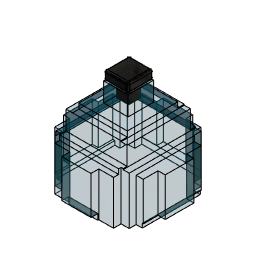
Sans nom v2 (Autodesk Fusion 360 design; units mm, degrees)
Autodesk Fusion 360 part; units mm, degrees
sketch "Esquisse1" plane through (0, 0, 0) normal (0, 0, 1) x (1, 0, 0)
  line L0 (25, 25) -> (-25, 25)
  line L1 (-25, 25) -> (-25, -25)
  line L2 (-25, -25) -> (25, -25)
  line L3 (25, -25) -> (25, 25)
  line L4 (25, 25) -> (-25, -25) construction
  line L5 (-25, 25) -> (25, -25) construction
  constraint horizontal L0
  constraint perpendicular L0 L1
  constraint parallel L0 L2
  constraint parallel L1 L3
  constraint coincident L4 origin
  constraint coincident L5 origin
sketch "Esquisse2" plane through (0, 0, 0) normal (0, 0, 1) x (1, 0, 0)
  line L0 (25, 0) -> (0, 0)
  line L1 (0, 0) -> (0, 25)
  line L2 (0, 25) -> (25, 25)
  line L3 (25, 25) -> (25, 0)
  line L4 (25, 9.1424) -> (0, 9.1424)
  line L5 (0, 9.1424) -> (0, 16.2)
  line L6 (0, 16.2) -> (25, 16.2)
  line L7 (25, 16.2) -> (25, 9.1424)
  line L8 (15.9, 0) -> (8.7089, 0)
  line L9 (8.7089, 0) -> (8.7089, 25)
  line L10 (8.7089, 25) -> (15.9, 25)
  line L11 (15.9, 25) -> (15.9, 0)
  line L12 (23.2024, 19.7988) -> (23.2024, 16.2)
  line L13 (19.595, 23.3399) -> (15.9, 23.3399)
  line L14 (23.2024, 19.7988) -> (21.4, 19.7988)
  line L15 (21.4, 19.7988) -> (21.4, 21.6)
  line L16 (21.4, 21.6) -> (19.57, 21.6)
  line L17 (19.57, 21.6) -> (19.595, 23.3399)
  line L18 (5.0893, 23.3546) -> (8.7089, 23.3546)
  line L19 (5.0893, 21.5398) -> (5.0893, 23.3546)
  line L20 (5.0893, 21.5398) -> (3.2612, 21.5398)
  line L21 (3.2612, 21.5398) -> (3.2612, 19.7651)
  line L22 (3.2612, 19.7651) -> (1.5, 19.7651)
  line L23 (1.5, 19.7651) -> (1.5, 16.2)
  line L24 (8.7089, 2.0063) -> (5, 2.0063)
  line L25 (5, 2.0063) -> (5, 3.7754)
  line L26 (5, 3.7754) -> (3.3188, 3.7754)
  line L27 (3.3188, 3.7754) -> (3.3188, 5.5)
  line L28 (3.3188, 5.5) -> (1.5, 5.5)
  line L29 (1.5, 5.5) -> (1.5, 9.1424)
  line L30 (15.9, 1.9294) -> (19.5, 1.9294)
  line L31 (19.5, 1.9294) -> (19.5, 3.7947)
  line L32 (19.5, 3.7947) -> (21.5, 3.7947)
  line L33 (21.5, 3.7947) -> (21.5, 5.5)
  line L34 (21.5, 5.5) -> (23.2404, 5.5)
  line L35 (23.2404, 5.5) -> (23.2404, 9.1424)
  constraint horizontal L0
  constraint vertical L1
  constraint horizontal L2
  constraint vertical L3
  constraint horizontal L4
  constraint vertical L5
  constraint horizontal L6
  constraint vertical L7
  constraint coincident L1 L5.end
  constraint coincident L3 L4.start
  constraint horizontal L8
  constraint vertical L9
  constraint horizontal L10
  constraint vertical L11
  constraint coincident L2 L9.end
  constraint coincident L0 L8.start
  constraint coincident L6 L12.end
  constraint perpendicular L6 L12
  constraint coincident L11 L13.end
  constraint perpendicular L11 L13
  constraint perpendicular L12 L14
  constraint perpendicular L14 L15
  constraint perpendicular L15 L16
  constraint coincident L9 L18.end
  constraint perpendicular L9 L18
  constraint perpendicular L18 L19
  constraint perpendicular L19 L20
  constraint perpendicular L20 L21
  constraint perpendicular L19 L22
  constraint coincident L6 L23.end
  constraint perpendicular L6 L23
  constraint coincident L9 L24.start
  constraint perpendicular L9 L24
  constraint perpendicular L24 L25
  constraint perpendicular L25 L26
  constraint perpendicular L26 L27
  constraint perpendicular L27 L28
  constraint coincident L4 L29.end
  constraint perpendicular L4 L29
  constraint coincident L11 L30.start
  constraint perpendicular L11 L30
  constraint perpendicular L30 L31
  constraint perpendicular L11 L32
  constraint perpendicular L32 L33
  constraint perpendicular L11 L34
  constraint coincident L4 L35.end
  constraint perpendicular L4 L35
extrude "Extrusion2" add sketch "Esquisse2" along normal blind 18 contours L0 L4 L8 L9 L11 | L3 L4 L6 L7 L11 | L4 L11 L30 L31 L32 L33 L34 L35 | L4 L9 L24 L25 L26 L27 L28 L29 | L4 L6 L9 L11 | L6 L11 L12 L13 L14 L15 L16 L17 | L1 L4 L5 L6 L9 | L2 L6 L9 L10 L11 | L6 L9 L18 L19 L20 L21 L22 L23 makes body 1
sketch "Esquisse3" plane through (0, 0, 0) normal (0, 1, 0) x (1, 0, 0)
  line L0 (25, -10.5) -> (21.5, -10.5)
  line L1 (21.5, -10.5) -> (21.5, -11.7872)
  line L2 (21.5, -11.7872) -> (20, -11.7872)
  line L3 (20, -11.7872) -> (20, -16.5)
  line L4 (20, -16.5) -> (18.5, -16.5)
  line L5 (18.5, -16.5) -> (18.5, -18)
  line L6 (18.5, -18) -> (15.5, -18)
  line L7 (15.5, -18) -> (15.5, -22.7294)
  line L8 (15.5, -22.7294) -> (14, -22.7294)
  line L9 (14, -22.7294) -> (14, -18)
  line L10 (14, -18) -> (15.5, -18)
  line L11 (-0.0186, -10.7584) -> (3.5, -10.7584)
  line L12 (3.5, -10.7584) -> (3.5, -11.8)
  line L13 (3.5, -11.8) -> (5, -11.8)
  line L14 (5, -11.8) -> (5, -16.7)
  line L15 (5, -16.7) -> (6.6, -16.7)
  line L16 (6.6, -16.7) -> (6.6, -18)
  line L17 (6.6, -18) -> (9.5, -18)
  line L18 (9.5, -18) -> (9.5, -22.7)
  line L19 (9.5, -22.7) -> (11.1, -22.7)
  line L20 (11.1, -22.7) -> (11.1, -18)
  line L21 (11.1, -18) -> (9.5, -18)
  line L22 (9.5, -22.7) -> (0, -22.7)
  line L23 (0, -22.7) -> (-0.0186, -10.7584)
  line L24 (15.5, -22.7294) -> (25, -22.7294)
  line L25 (25, -22.7294) -> (25, -10.5)
  constraint horizontal L0
  constraint perpendicular L0 L1
  constraint perpendicular L1 L2
  constraint perpendicular L2 L3
  constraint perpendicular L3 L4
  constraint perpendicular L4 L5
  constraint perpendicular L5 L6
  constraint perpendicular L6 L7
  constraint perpendicular L7 L8
  constraint perpendicular L8 L9
  constraint perpendicular L7 L10
  constraint horizontal L11
  constraint perpendicular L11 L12
  constraint perpendicular L12 L13
  constraint perpendicular L11 L14
  constraint perpendicular L14 L15
  constraint perpendicular L15 L16
  constraint perpendicular L16 L17
  constraint perpendicular L17 L18
  constraint perpendicular L18 L19
  constraint perpendicular L19 L20
  constraint perpendicular L18 L21
  constraint perpendicular L18 L22
  constraint perpendicular L7 L24
  constraint perpendicular L0 L25
extrude "Extrusion3" cut sketch "Esquisse3" along normal blind 39 contours L0 L1 L2 L3 L4 L5 L6 L7 L24 L25 | L11 L12 L13 L14 L15 L16 L17 L18 L22 L23 bodies 1
sketch "Esquisse4" plane through (0, 25, 0) normal (0, 1, 0) x (-1, 0, 0)
  line L0 (-15.9, 0) -> (-8.7089, 0)
  line L1 (-8.7089, 0) -> (-8.7089, 18)
  line L2 (-8.7089, 18) -> (-15.9, 18)
  line L3 (-15.9, 18) -> (-15.9, 0)
  line L4 (-25, 1) -> (-23, 1)
  line L5 (-23, 1) -> (-23, -0.7028)
  line L6 (-23, -0.7028) -> (-25, -0.7028)
  line L7 (-25, -0.7028) -> (-25, 1)
  line L8 (-2, 1) -> (1, 1)
  line L9 (1, 1) -> (1, -1.75)
  line L10 (1, -1.75) -> (-2, -1.75)
  line L11 (-2, -1.75) -> (-2, 1)
  constraint horizontal L4
  constraint perpendicular L4 L5
  constraint perpendicular L5 L6
  constraint perpendicular L4 L7
  constraint perpendicular L7 L8
  constraint perpendicular L8 L9
  constraint perpendicular L9 L10
  constraint perpendicular L8 L11
extrude "Extrusion4" cut sketch "Esquisse4" against normal blind 27 contours L4 L5 L6 L7 | L8 L9 L10 L11 bodies 1
sketch "Esquisse5" plane through (25, 0, 0) normal (1, 0, 0) x (0, 1, 0)
  line L0 (9.1424, 1) -> (16.2, 1)
  line L1 (16.2, 1) -> (16.2, 10.5)
  line L2 (16.2, 10.5) -> (9.1424, 10.5)
  line L3 (9.1424, 10.5) -> (9.1424, 1)
  line L4 (-0.1313, 10.8245) -> (28, 10.8245)
  line L5 (28, 10.8245) -> (28, 18)
  line L6 (28, 18) -> (-0.1313, 18)
  line L7 (-0.1313, 18) -> (-0.1313, 10.8245)
  line L8 (3.1847, 10.8245) -> (-0.1313, 10.8245)
  line L9 (-0.1313, 10.8245) -> (-0.1313, 18)
  line L10 (-0.1313, 18) -> (3.1847, 18)
  line L11 (3.1847, 18) -> (3.1847, 10.8245)
  line L12 (4.7584, 12.0208) -> (3.1847, 12.0208)
  line L13 (3.1847, 12.0208) -> (3.1847, 18)
  line L14 (3.1847, 18) -> (4.7584, 18)
  line L15 (4.7584, 18) -> (4.7584, 12.0208)
  line L16 (6.3321, 16.7068) -> (4.7584, 16.7068)
  line L17 (4.7584, 16.7068) -> (4.7584, 18)
  line L18 (4.7584, 18) -> (6.3321, 18)
  line L19 (6.3321, 18) -> (6.3321, 16.7068)
  line L20 (18.7115, 18) -> (28, 18)
  line L21 (28, 18) -> (28, 16.7068)
  line L22 (28, 16.7068) -> (18.7115, 16.7068)
  line L23 (18.7115, 16.7068) -> (18.7115, 18)
  line L24 (20.3201, 16.7068) -> (28, 16.7068)
  line L25 (28, 16.7068) -> (28, 12)
  line L26 (28, 12) -> (20.3201, 12)
  line L27 (20.3201, 12) -> (20.3201, 16.7068)
  line L28 (28, 10.8245) -> (21.8, 10.8245)
  line L29 (21.8, 10.8245) -> (21.8, 12)
  line L30 (21.8, 12) -> (28, 12)
  line L31 (28, 12) -> (28, 10.8245)
  constraint horizontal L4
  constraint vertical L5
  constraint horizontal L6
  constraint vertical L7
  constraint horizontal L8
  constraint vertical L9
  constraint horizontal L10
  constraint vertical L11
  constraint coincident L4 L8.start
  constraint horizontal L12
  constraint vertical L13
  constraint horizontal L14
  constraint vertical L15
  constraint horizontal L16
  constraint vertical L17
  constraint horizontal L18
  constraint vertical L19
  constraint horizontal L20
  constraint vertical L21
  constraint horizontal L22
  constraint vertical L23
  constraint coincident L5 L21.end
  constraint coincident L6 L20.start
  constraint horizontal L24
  constraint vertical L25
  constraint horizontal L26
  constraint vertical L27
  constraint coincident L5 L25.end
  constraint coincident L22 L24.start
  constraint horizontal L28
  constraint vertical L29
  constraint horizontal L30
  constraint vertical L31
  constraint coincident L26 L29.end
extrude "Extrusion5" cut sketch "Esquisse5" against normal blind 32 contours L4 L6 L7 L8 L9 L10 L11 L13 | L4 L5 L26 L28 L29 L30 L31 | L6 L11 L12 L13 L14 L15 L17 | L5 L22 L24 L25 L26 L27 L30 | L6 L15 L16 L17 L18 L19 | L5 L6 L20 L21 L22 L23 L24 bodies 1
sketch "Esquisse6" plane through (25, 0, 0) normal (1, 0, 0) x (0, 1, 0)
  line L0 (9.1424, 1) -> (16.2, 1)
  line L1 (16.2, 1) -> (16.2, 10.5)
  line L2 (16.2, 10.5) -> (9.1424, 10.5)
  line L3 (9.1424, 10.5) -> (9.1424, 1)
  line L4 (23.3, 1.5) -> (25.7, 1.5)
  line L5 (25.7, 1.5) -> (25.7, -0.6)
  line L6 (25.7, -0.6) -> (23.3, -0.6)
  line L7 (23.3, -0.6) -> (23.3, 1.5)
  line L8 (1.7, 1.45) -> (-0.9, 1.45)
  line L9 (-0.9, 1.45) -> (-0.9, -0.6)
  line L10 (-0.9, -0.6) -> (1.7, -0.6)
  line L11 (1.7, -0.6) -> (1.7, 1.45)
  constraint horizontal L4
  constraint vertical L5
  constraint horizontal L6
  constraint vertical L7
  constraint horizontal L8
  constraint vertical L9
  constraint horizontal L10
  constraint vertical L11
extrude "Extrusion6" cut sketch "Esquisse6" against normal blind 26 contours L4 L5 L6 L7 | L8 L9 L10 L11 bodies 1
sketch "Esquisse7" plane through (0, 0, 18) normal (0, 0, 1) x (-1, 0, 0)
  line L0 (-6.6, -6.3321) -> (-18.5, -6.3321)
  line L1 (-18.5, -6.3321) -> (-18.5, -18.7115)
  line L2 (-18.5, -18.7115) -> (-6.6, -18.7115)
  line L3 (-6.6, -18.7115) -> (-6.6, -6.3321)
  line L4 (-15, -10) -> (-10, -10)
  line L5 (-10, -10) -> (-10, -15)
  line L6 (-10, -15) -> (-15, -15)
  line L7 (-15, -15) -> (-15, -10)
  constraint horizontal L4
  constraint vertical L5
  constraint horizontal L6
  constraint vertical L7
extrude "Extrusion7" add sketch "Esquisse7" along normal blind 7 contours L4 L5 L6 L7 bodies 1
extrude "Extrusion8" add 1 faces at (10, 11.6667, 20.3333) along direction (-1, 0, 0) blind 0.4 on bodies 1 bodies 1
extrude "Extrusion9" add 1 faces at (15, 13.3333, 20.3333) along direction (1, 0, 0) blind 0.6 on bodies 1 bodies 1
extrude "Extrusion10" add 1 faces at (13.6, 15, 20.3333) along direction (0, 1, 0) blind 0.7 on bodies 1 bodies 1
extrude "Extrusion11" add 1 faces at (11.6, 10, 20.3333) along direction (0, -1, 0) blind 0.6 on bodies 1 bodies 1
sketch "Esquisse8" plane through (0, 0, 25) normal (0, 0, 1) x (-1, 0, 0)
  line L0 (-9.6, -15.7) -> (-9.6, -9.4)
  line L1 (-9.6, -9.4) -> (-15.6, -9.4)
  line L2 (-15.6, -9.4) -> (-15.6, -15.7)
  line L3 (-15.6, -15.7) -> (-9.6, -15.7)
  line L4 (-15.0873, -15.2195) -> (-10.1127, -15.2195)
  line L5 (-10.1127, -15.2195) -> (-10.1127, -9.8805)
  line L6 (-10.1127, -9.8805) -> (-15.0873, -9.8805)
  line L7 (-15.0873, -9.8805) -> (-15.0873, -15.2195)
  line L8 (-15.0873, -15.2195) -> (-10.1127, -9.8805) construction
  point P0 (-12.6, -12.55)
  constraint horizontal L4
  constraint perpendicular L4 L5
  constraint parallel L4 L6
  constraint parallel L5 L7
  constraint coincident L8 P0
extrude "Extrusion12" cut sketch "Esquisse8" against normal blind 6 contours L4 L5 L6 L7 bodies 1
extrude "Extrusion13" add 1 faces at (13.4291, 15.2195, 23) along direction (0, -1, 0) blind 1.2 on bodies 1 bodies 1
extrude "Extrusion14" add 1 faces at (11.7709, 9.8805, 23) along direction (0, 1, 0) blind 1.2 on bodies 1 bodies 1
extrude "Extrusion15" add 1 faces at (15.0873, 12.0602, 23) along direction (-1, 0, 0) blind 1 on bodies 1 bodies 1
extrude "Extrusion16" add 1 faces at (10.1127, 13.0398, 23) along direction (1, 0, 0) blind 1 on bodies 1 bodies 1
extrude "Extrusion17" cut 1 faces at (12.1042, 15.1398, 25) along direction (0, 0, -1) blind 2.3 on bodies 1 bodies 1
extrude "Extrusion18" add 1 faces at (12.1042, 12.0602, 19) along direction (0, 0, 1) blind 3.7 separate body on bodies 1 makes body 2
extrude "Extrusion19" add 2 faces at (12.1042, 15.1398, 22.7) (12.1042, 12.0602, 22.7) along direction (0, 0, 1) blind 2.4 separate body on bodies 1 2 makes body 3
fillet "Congé1" radius 0.5 12 edges at (12.6, 9.4, 25.1) (9.6, 12.55, 25.1) (15.6, 12.55, 25.1) (12.6, 15.7, 25.1) (9.6, 12.55, 22.7) (12.6, 15.7, 22.7) (15.6, 12.55, 22.7) (12.6, 9.4, 22.7) (15.6, 9.4, 23.9) (9.6, 9.4, 23.9) (9.6, 15.7, 23.9) (15.6, 15.7, 23.9) on bodies 3
combine "Combiner1" operation add target body 3 tool bodies 2
sketch "Esquisse9" plane through (0, 0, 0) normal (0, 0, 1) x (1, 0, 0)
  line L0 (-15, -15) -> (-25, -15)
  line L1 (-25, -15) -> (-25, -25)
  line L2 (-25, -25) -> (-15, -25)
  line L3 (-15, -25) -> (-15, -15)
  constraint horizontal L0
  constraint vertical L1
  constraint horizontal L2
  constraint vertical L3
sketch "Esquisse10" plane through (0, 0, 2.5) normal (0, 0, 1) x (-1, 0, 0)
  line L0 (15, 25) -> (15, 15)
  line L1 (15, 15) -> (25, 15)
  line L2 (25, 15) -> (25, 25)
  line L3 (25, 25) -> (15, 25)
  line L4 (10, 10) -> (30, 10)
  line L5 (30, 10) -> (30, 30)
  line L6 (30, 30) -> (10, 30)
  line L7 (10, 30) -> (10, 10)
  line L8 (10, 10) -> (30, 30) construction
  line L9 (30, 10) -> (10, 30) construction
  point P0 (20, 20)
  constraint horizontal L4
  constraint perpendicular L4 L5
  constraint parallel L4 L6
  constraint parallel L5 L7
  constraint coincident L8 P0
  constraint coincident L9 P0
sketch "Esquisse11" plane through (0, 0, 5) normal (0, 0, 1) x (-1, 0, 0)
  line L0 (15, 25) -> (25, 25)
  line L1 (25, 25) -> (25, 15)
  line L2 (25, 15) -> (15, 15)
  line L3 (15, 15) -> (15, 25)
  line L4 (10, 30) -> (10, 10)
  line L5 (10, 10) -> (30, 10)
  line L6 (30, 10) -> (30, 30)
  line L7 (30, 30) -> (10, 30)
  line L8 (7, 7) -> (33, 7)
  line L9 (33, 7) -> (33, 33)
  line L10 (33, 33) -> (7, 33)
  line L11 (7, 33) -> (7, 7)
  line L12 (7, 7) -> (33, 33) construction
  line L13 (33, 7) -> (7, 33) construction
  point P0 (20, 20)
  constraint horizontal L8
  constraint perpendicular L8 L9
  constraint parallel L8 L10
  constraint parallel L9 L11
  constraint coincident L12 P0
  constraint coincident L13 P0
sketch "Esquisse12" plane through (-7, 0, 0) normal (1, 0, 0) x (0, 1, 0)
  line L0 (-7, 7.5) -> (-7, 26.5)
  line L1 (-7, 26.5) -> (-33, 26.5)
  line L2 (-33, 26.5) -> (-33, 7.5)
  line L3 (-33, 7.5) -> (-7, 7.5)
sketch "Esquisse13" plane through (0, 0, 26.5) normal (0, 0, 1) x (-1, 0, 0)
  line L0 (10, 30) -> (30, 30)
  line L1 (30, 30) -> (30, 10)
  line L2 (30, 10) -> (10, 10)
  line L3 (10, 10) -> (10, 30)
  line L4 (7, 33) -> (7, 7)
  line L5 (7, 7) -> (33, 7)
  line L6 (33, 7) -> (33, 33)
  line L7 (33, 33) -> (7, 33)
  circle A0 centre (20, 20) radius 13
  constraint tangent L4 A0
